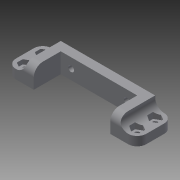
# Autodesk Inventor part: WALLY MOUNT
Saved by Autodesk Inventor 2013 (Build 170138000, 138)
## iProperties
Created: 2014-01-04
Part Number: WALLY MOUNT
Material: Generic
Document SubType Name: Modeling
Designer: employee
Density: 1 g/cm^3
Author: employee
Autodesk Inventor part; units mm, degrees
ref_plane "YZ Plane" through (0, 0, 0) normal (1, 0, 0) x (0, 1, 0)
ref_plane "XZ Plane" through (0, 0, 0) normal (0, 1, 0) x (-1, 0, 0)
ref_plane "XY Plane" through (0, 0, 0) normal (0, 0, 1) x (1, 0, 0)
sketch "Sketch1" plane through (0, 0, 0) normal (0, 0, 1) x (1, 0, 0)
  line L0 (-36.25, -15) -> (-21.25, -15)
  line L1 (-21.25, -15) -> (-21.25, 0)
  line L2 (-21.25, 0) -> (21.25, 0)
  line L3 (21.25, 0) -> (21.25, -15)
  line L4 (21.25, -15) -> (36.25, -15)
  line L5 (36.25, -15) -> (36.25, 5)
  line L6 (36.25, 5) -> (-36.25, 5)
  line L7 (-36.25, 5) -> (-36.25, -15)
  point P0 (0, 0)
  point P1 (0, 0)
  dimension "d0" = 42.5
  dimension "d2" = 20
  dimension "d3" = 15
  dimension "d4" = 5
  constraints: 16 end point, 5 parallel, 2 equal length, 2 horizontal, 1 coincident, 1 midpoint, 1 perpendicular
  measures "d0" distance of L1.end L2.end
  measures "d2" distance of L6.end L0.start
  measures "d3" distance of L0.start L0.end
  measures "d4" distance between parallel lines of L6 L2
extrude "Extrusion1" add sketch "Sketch1" along normal blind 5
sketch "Sketch2" plane through (0, 0, 5) normal (0, 0, 1) x (1, 0, 0)
  line L0 (-36.25, -15) -> (-21.25, -15) projected
  line L1 (-21.25, -15) -> (-21.25, 0) projected
  line L2 (-21.25, 0) -> (21.25, 0) projected
  line L3 (21.25, 0) -> (21.25, -15) projected
  line L4 (36.25, 5) -> (-36.25, 5) projected
  line L5 (-36.25, 5) -> (-36.25, -15) projected
  line L6 (-26.25, 5) -> (-26.25, -15)
  line L7 (26.25, -15) -> (26.25, 5)
  line L8 (-26.25, 5) -> (26.25, 5)
  line L9 (26.25, -15) -> (21.25, -15)
  line L10 (-26.25, -15) -> (-21.25, -15)
  point P0 (0, 0)
  dimension "d7" = 5
  dimension "d8" = 5
  constraints: 10 end point, 3 point on line, 2 perpendicular, 1 collinear, 1 horizontal, 1 parallel
  measures "d7" distance between parallel lines of L3 L7
  measures "d8" distance between parallel lines of L1 L6
extrude "Extrusion2" add sketch "Sketch2" along normal blind 6 contours L6 L4 L7 L9 L3 L2 L1 L0
sketch "Sketch3" plane through (0, 0, 5) normal (0, 0, 1) x (1, 0, 0)
  line L0 (-26.25, 5) -> (-36.25, 5) projected
  line L1 (-36.25, 5) -> (-36.25, -15) projected
  line L2 (26.25, 5) -> (26.25, -15) projected
  line L3 (26.25, -15) -> (36.25, -15) projected
  line L4 (36.25, -15) -> (36.25, 5) projected
  line L5 (36.25, 5) -> (26.25, 5) projected
  line L6 (-31.25, 0) -> (31.25, 0)
  line L7 (31.25, 0) -> (31.25, -10)
  line L8 (31.25, -10) -> (-31.25, -10)
  line L9 (-31.25, -10) -> (-31.25, 0)
  line L10 (-21.25, 0) -> (21.25, 0) projected
  circle A0 centre (-31.25, 0) radius 1.6
  circle A1 centre (-31.25, -10) radius 1.6
  circle A2 centre (31.25, -10) radius 1.6
  circle A3 centre (31.25, 0) radius 1.6
  point P0 (0, 0)
  point P1 (-31.25, -5)
  point P2 (-36.25, -5)
  point P3 (0, -10)
  point P4 (0, 0)
  point P5 (-31.25, 5)
  dimension "d11" = 10
  dimension "d13" = 3.2
  constraints: 8 end point, 5 midpoint, 4 centre point, 4 coincident, 3 equal radius, 2 parallel, 2 vertical alignment, 1 horizontal, 1 horizontal alignment, 1 perpendicular
  measures "d11" distance of L8.end L6.start
  measures "d13" diameter of A3
extrude "Extrusion3" cut sketch "Sketch3" against normal blind 5 contours A3 L7 L6 | L6 L7 A3 | A2 L7 L8 | L8 L7 A2 | A1 L9 L8 | L8 L9 A1 | A0 L9 L6 | L6 L9 A0
sketch "Sketch4" plane through (0, 0, 5) normal (0, 0, 1) x (1, 0, 0)
  circle A0 centre (-31.25, -10) radius 1.6 projected
  circle A1 centre (-31.25, 0) radius 1.6 projected
  circle A2 centre (31.25, 0) radius 1.6 projected
  circle A3 centre (31.25, -10) radius 1.6 projected
  line L0 (26.25, 5) -> (26.25, -15) projected
  line L1 (26.25, -15) -> (36.25, -15) projected
  line L2 (36.25, -15) -> (36.25, 5) projected
  line L3 (36.25, 5) -> (26.25, 5) projected
  line L4 (-31.25, -3.2332) -> (-34.05, -1.6166)
  line L5 (-34.05, -1.6166) -> (-34.05, 1.6166)
  line L6 (-34.05, 1.6166) -> (-31.25, 3.2332)
  line L7 (-31.25, 3.2332) -> (-28.45, 1.6166)
  line L8 (-28.45, 1.6166) -> (-28.45, -1.6166)
  line L9 (-28.45, -1.6166) -> (-31.25, -3.2332)
  line L10 (-31.25, -6.7668) -> (-28.45, -8.3834)
  line L11 (-28.45, -8.3834) -> (-28.45, -11.6166)
  line L12 (-28.45, -11.6166) -> (-31.25, -13.2332)
  line L13 (-31.25, -13.2332) -> (-34.05, -11.6166)
  line L14 (-34.05, -11.6166) -> (-34.05, -8.3834)
  line L15 (-34.05, -8.3834) -> (-31.25, -6.7668)
  line L16 (31.25, -6.7668) -> (34.05, -8.3834)
  line L17 (34.05, -8.3834) -> (34.05, -11.6166)
  line L18 (34.05, -11.6166) -> (31.25, -13.2332)
  line L19 (31.25, -13.2332) -> (28.45, -11.6166)
  line L20 (28.45, -11.6166) -> (28.45, -8.3834)
  line L21 (28.45, -8.3834) -> (31.25, -6.7668)
  line L22 (31.25, 3.2332) -> (34.05, 1.6166)
  line L23 (34.05, 1.6166) -> (34.05, -1.6166)
  line L24 (34.05, -1.6166) -> (31.25, -3.2332)
  line L25 (31.25, -3.2332) -> (28.45, -1.6166)
  line L26 (28.45, -1.6166) -> (28.45, 1.6166)
  line L27 (28.45, 1.6166) -> (31.25, 3.2332)
  point P0 (0, 0)
  dimension "d16" = 5.6
  constraints: 48 end point, 4 coincident, 4 vertical, 3 equal length, 52 other
  measures "d16" distance between parallel lines of L26 L23
extrude "Extrusion4" cut sketch "Sketch4" against normal blind 2.5 contours L4 L5 L6 L7 L8 L9 | L10 L11 L12 L13 L14 L15 | L16 L17 L18 L19 L20 L21 | L22 L23 L24 L25 L26 L27
fillet "Fillet1" radius 5 8 edges at (-26.25, -5, 5) (-36.25, -15, 2.5) (-36.25, 5, 2.5) (26.25, -5, 5) (36.25, -15, 2.5) (36.25, 5, 2.5) (-23.75, -15, 11) (23.75, -15, 11)
sketch "Sketch5" plane through (-26.25, 5, 11) normal (0, 1, 0) x (1, 0, 0)
  line L0 (57.5, 11) -> (-5, 11) projected
  line L1 (5.25, 11) -> (47.25, 11)
  line L2 (47.25, 11) -> (47.25, -31)
  line L3 (47.25, -31) -> (5.25, -31)
  line L4 (5.25, -31) -> (5.25, 11)
  line L5 (10.75, 5.5) -> (41.75, 5.5)
  line L6 (41.75, 5.5) -> (41.75, -25.5)
  line L7 (41.75, -25.5) -> (10.75, -25.5)
  line L8 (10.75, -25.5) -> (10.75, 5.5)
  circle A0 centre (10.75, 5.5) radius 1.6
  circle A1 centre (41.75, 5.5) radius 1.6
  point P0 (26.25, 11)
  point P1 (26.25, 11)
  point P2 (41.75, -10)
  point P3 (47.25, -10)
  point P4 (26.25, 5.5)
  point P5 (26.25, 11)
  dimension "d20" = 42
  dimension "d22" = 31
  dimension "d23" = 3.2
  constraints: 16 end point, 6 midpoint, 4 parallel, 4 perpendicular, 2 centre point, 2 coincident, 2 horizontal, 1 equal radius, 1 horizontal alignment, 1 vertical alignment
  measures "d20" distance of L1.end L2.end
  measures "d22" distance of L5.start L5.end
  measures "d23" diameter of A1
extrude "Extrusion5" cut sketch "Sketch5" against normal through all contours L8 A0 L5 | L5 A0 L8 | A1 L6 L5 | L5 L6 A1
body "Solid1"
